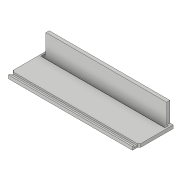
# Autodesk Inventor part: Electronics Container Part 5
Saved by Autodesk Inventor 2018.3 (Build 223284000, 284)
## iProperties
Created: 2019-03-04
Part Number: Electronics Container Part 5
Material: Generic
Document SubType Name: Modeling
Designer: aye06091
Mass: 20.094 g
Surface Area: 153.494 cm^2
Volume: 20.094 cm^3
Density: 1 g/cm^3
Appearance: Default
Author: aye06091
Autodesk Inventor part; units mm, degrees
ref_plane "YZ Plane" through (0, 0, 0) normal (1, 0, 0) x (0, 1, 0)
ref_plane "XZ Plane" through (0, 0, 0) normal (0, 1, 0) x (-1, 0, 0)
ref_plane "XY Plane" through (0, 0, 0) normal (0, 0, 1) x (1, 0, 0)
sketch "Sketch1" plane through (0, 0, 0) normal (0, 1, 0) x (-1, 0, 0)
  line L0 (0, 0) -> (-123.825, 0)
  line L1 (-123.825, 0) -> (-123.825, 38.1)
  line L2 (-123.825, 38.1) -> (0, 38.1)
  line L3 (0, 38.1) -> (0, 0)
  dimension "d0" = 123.825
  dimension "d1" = 38.1
  constraints: 8 end point, 2 parallel, 1 horizontal, 1 perpendicular
  measures "d0" distance of L0.start L0.end
  measures "d1" distance of L0.end L1.end
extrude "Extrusion1" add sketch "Sketch1" along normal blind 3.175
sketch "Sketch2" plane through (0, 3.175, 0) normal (0, 1, 0) x (1, 0, 0)
  line L0 (123.825, 0) -> (0, 0) projected
  line L1 (0, 0) -> (0, -38.1) projected
  line L2 (0, -38.1) -> (123.825, -38.1) projected
  line L3 (123.825, -38.1) -> (123.825, 0) projected
  line L4 (0, -36.5125) -> (123.825, -36.5125)
  line L5 (123.825, -36.5125) -> (123.825, -33.3121)
  line L6 (123.825, -33.3121) -> (0, -33.3121)
  line L7 (0, -33.3121) -> (0, -36.5125)
  line L8 (1.5875, -3.175) -> (87.3125, -3.175)
  line L9 (87.3125, -3.175) -> (87.3125, -6.604)
  line L10 (87.3125, -6.604) -> (1.5875, -6.604)
  line L11 (1.5875, -6.604) -> (1.5875, -3.175)
  dimension "d4" = 3.2004
  dimension "d5" = 1.5875
  dimension "d8" = 85.725
  dimension "d9" = 1.5875
  dimension "d10" = 3.429
  dimension "d11" = 3.175
  constraints: 16 end point, 4 parallel, 2 horizontal, 2 perpendicular, 2 point on line
  measures "d4" distance between parallel lines of L4 L6
  measures "d5" distance between parallel lines of L2 L4
  measures "d8" distance of L8.start L8.end
  measures "d9" distance between parallel lines of L1 L11
  measures "d10" distance between parallel lines of L8 L10
  measures "d11" distance between parallel lines of L0 L8
extrude "Extrusion2" cut sketch "Sketch2" against normal blind 1.5875 contours L3 L4 L1 L6
sketch "Sketch3" plane through (0, 3.175, 0) normal (0, 1, 0) x (1, 0, 0)
  line L0 (123.825, 0) -> (0, 0) projected
  line L1 (0, 0) -> (0, -33.3121) projected
  line L2 (1.5875, -3.175) -> (122.2375, -3.175)
  line L3 (122.2375, -3.175) -> (122.2375, -6.604)
  line L4 (122.2375, -6.604) -> (1.5875, -6.604)
  line L5 (1.5875, -6.604) -> (1.5875, -3.175)
  line L6 (123.825, -33.3121) -> (123.825, 0) projected
  dimension "d15" = 3.429
  dimension "d16" = 3.175
  dimension "d17" = 1.5875
  dimension "d20" = 1.5875
  constraints: 8 end point, 2 parallel, 1 horizontal, 1 perpendicular
  measures "d15" distance between parallel lines of L2 L4
  measures "d16" distance between parallel lines of L0 L2
  measures "d17" distance between parallel lines of L1 L5
  measures "d20" distance between parallel lines of L6 L3
extrude "Extrusion3" cut sketch "Sketch3" against normal blind 12.7
sketch "Sketch4" plane through (0, 3.175, 0) normal (0, 1, 0) x (1, 0, 0)
  line L0 (0, -38.1) -> (1.5875, -38.1)
  line L1 (1.5875, -38.1) -> (1.5875, -31.75)
  line L2 (1.5875, -31.75) -> (0, -31.75)
  line L3 (0, -31.75) -> (0, -38.1)
  line L4 (123.825, -38.1) -> (122.2375, -38.1)
  line L5 (122.2375, -38.1) -> (122.2375, -31.75)
  line L6 (122.2375, -31.75) -> (123.825, -31.75)
  line L7 (123.825, -31.75) -> (123.825, -38.1)
  point P0 (0, 0)
  dimension "d21" = 1.5875
  dimension "d22" = 6.35
  dimension "d23" = 6.35
  dimension "d24" = 1.5875
  constraints: 16 end point, 4 parallel, 2 horizontal, 2 perpendicular, 1 point on line
  measures "d21" distance between parallel lines of L3 L1
  measures "d22" distance of L0.end L1.end
  measures "d23" distance of L4.end L5.end
  measures "d24" distance of L5.end L6.end
extrude "Extrusion4" cut sketch "Sketch4" against normal blind 12.7
fillet "Fillet1" radius 1.5875 2 edges at (122.2375, 1.5875, 31.75) (1.5875, 1.5875, 31.75)
sketch "Sketch5" plane through (0, 3.175, 0) normal (0, 1, 0) x (1, 0, 0)
  line L0 (123.825, -31.75) -> (123.825, 0) projected
  line L1 (3.2004, 0) -> (120.6246, 0)
  line L2 (120.6246, 0) -> (120.6246, -3.175)
  line L3 (120.6246, -3.175) -> (3.2004, -3.175)
  line L4 (3.2004, -3.175) -> (3.2004, 0)
  line L5 (0, 0) -> (0, -31.75) projected
  dimension "d31" = 3.175
  dimension "d32" = 3.2004
  dimension "d33" = 3.2004
  constraints: 8 end point, 2 parallel, 1 horizontal, 1 perpendicular
  measures "d31" distance between parallel lines of L1 L3
  measures "d32" distance between parallel lines of L0 L2
  measures "d33" distance between parallel lines of L5 L4
extrude "Extrusion5" add sketch "Sketch5" along normal blind 19.05
body "Solid1"
